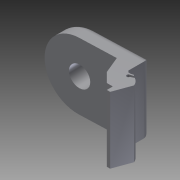
# Autodesk Inventor part: PiedClip
Saved by Autodesk Inventor 2012 (Build 160160000, 160)
## iProperties
Created: 2013-03-12
Part Number: PiedClip
Material: Default
Document SubType Name: Modeling
Designer: mce
Density: 1 g/cm^3
Author: mce
Autodesk Inventor part; units mm, degrees
ref_plane "YZ Plane" through (0, 0, 0) normal (1, 0, 0) x (0, 1, 0)
ref_plane "XZ Plane" through (0, 0, 0) normal (0, 1, 0) x (-1, 0, 0)
ref_plane "XY Plane" through (0, 0, 0) normal (0, 0, 1) x (1, 0, 0)
sketch "Sketch1" plane through (0, 0, 0) normal (0, 0, 1) x (1, 0, 0)
  line L0 (0, 0) -> (20.9872, 0.7329)
  line L1 (20.9872, 0.7329) -> (20.9872, -7.2671)
  line L2 (20.9872, -7.2671) -> (27.7872, -7.2671)
  line L3 (27.7872, -7.2671) -> (27.7872, -9.0671)
  line L4 (27.1872, -1.2671) -> (25.9872, -1.2671)
  line L5 (25.9872, -1.2671) -> (25.9872, 5.9105)
  line L6 (25.9872, 5.9105) -> (0, 5.003)
  line L7 (0, 5.003) -> (0, 0)
  line L8 (30.7063, -3.7945) -> (28.7872, -9.0671)
  line L9 (28.7872, -9.0671) -> (27.7872, -9.0671)
  line L10 (27.1872, -1.2671) -> (27.8551, -1.0596)
  line L11 (27.8551, -1.0596) -> (28.2648, -1.3511)
  line L12 (28.2648, -1.3511) -> (27.2091, -1.6792)
  arc A0 (30.7063, -3.7945) -> (28.8522, -1.7285) centre (26.9872, -5.2671) ccw
  arc A1 (27.2091, -1.6792) -> (27.8551, -2.2058) centre (27.3575, -2.1566) ccw
  line L13 (27.8551, -2.2058) -> (28.8522, -1.7285)
  point P0 (30.7872, -1.2671)
  dimension "d0" = 21
  dimension "d1" = 5
  dimension "d2" = 5
  dimension "d4" = 1.8
  dimension "d5" = 6
  dimension "d6" = 1.8
  dimension "d31" = 88
  dimension "d32" = 8
  dimension "d35" = 110
  dimension "d36" = 1
  dimension "d38" = 6
  dimension "d40" = 0.4
  dimension "d41" = 4
  dimension "d42" = 2
  dimension "d44" = 1.2
  dimension "d45" = 1
  constraints: 28 end point, 4 point on circle, 2 centre point, 2 perpendicular, 2 vertical, 1 equal length, 1 point on line, 1 tangent
  measures "d0" distance of L0.start L0.end
  measures "d1" distance between parallel lines of L6 L0
  measures "d2" distance between parallel lines of L1 L5
  measures "d4" distance between parallel lines of L5 L3
  measures "d5" distance between parallel lines of L4 L2
  measures "d6" distance of L2.end L3.end
  measures "d31" angle of L0 L1
  measures "d32" distance from line of L0.end L2
  measures "d35" angle of L8 L9
  measures "d36" distance of L8.end L3.end
  measures "d38" distance from line of L1 A0.centre
  measures "d40" distance between parallel lines of L10 L12
  measures "d41" radius of A0
  measures "d42" distance from line of L2 A0.centre
  measures "d44" distance of L4.start L4.end
  measures "d45" diameter of A1
extrude "Extrusion1" add sketch "Sketch1" along normal blind 20
fillet "Fillet1" [suppressed]
fillet "Fillet2" radius 10 2 edges at (0, 2.5015, 0) (0, 2.5015, 20)
sketch "Sketch2" plane through (10, 5.3523, 10) normal (-0.0349, 0.9994, 0) x (0, 0, -1)
  circle A0 centre (0, 0) radius 3.1
  ellipse E0 centre (0, 0) end of major axis (0, 10.0061) minor radius 10 (10, 0) -> (-10, 0) ccw projected
  line L0 (-10, 0) -> (-10, -15.997) projected
  point P0 (10, 10.1807)
  dimension "d16" = 6.2
  dimension "d33" = 10
  dimension "d34" = 0
  constraints: 1 centre point, 1 other
  measures "d16" diameter of A0
  measures "d33" distance from line of L0 A0.centre
  measures "d34" distance of point (0, 0) A0.centre
extrude "Extrusion2" cut sketch "Sketch2" against normal blind 10
fillet "Fillet3" radius 2 4 edges at (17.9934, 5.6314, 0) (2.9288, 5.1053, 2.9288) (17.9934, 5.6314, 20) (25.9872, 5.9105, 10)
chamfer "Chamfer2" distance 5 angle 45 1 edges at (20.9872, -7.2671, 10)
chamfer "Chamfer3" distance 3 angle 45 1 edges at (20.9872, -2.2671, 10)
chamfer "Chamfer4" distance 0.5 angle 45 1 edges at (25.9872, -1.2671, 10)
body "Solid1"
